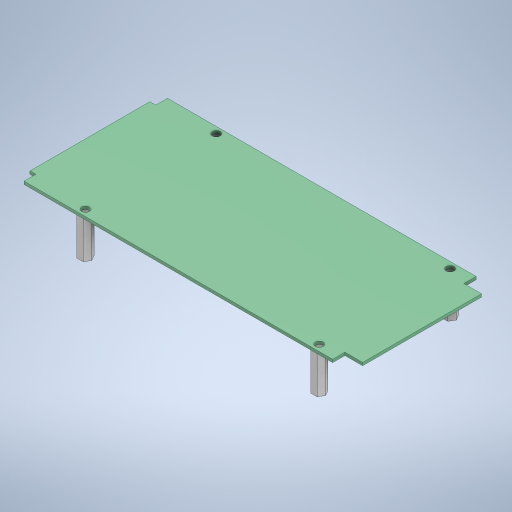
# Autodesk Inventor part: Tarjeta IC DC
Saved by Autodesk Inventor 2024.2 (Build 282272000, 272)
## iProperties
Created: 2024-08-27
Part Number: Tarjeta IC DC
Material: Phenolic Resin
Document SubType Name: Modeling
Designer: ja.restrepo1
Density: 1.38 g/cm^3
Appearance: Smooth - Dark Sea Green
Author: ja.restrepo1
Autodesk Inventor part; units mm, degrees
ref_plane "YZ Plane" through (0, 0, 0) normal (1, 0, 0) x (0, 1, 0)
ref_plane "XZ Plane" through (0, 0, 0) normal (0, 1, 0) x (-1, 0, 0)
ref_plane "XY Plane" through (0, 0, 0) normal (0, 0, 1) x (1, 0, 0)
sketch "Sketch1" plane through (0, 0, 0) normal (0, 1, 0) x (-1, 0, 0)
  line L0 (81.5, 36.5) -> (78.5, 36.5) construction
  line L1 (-78.5, 36.5) -> (-78.5, 30.25)
  line L2 (-78.5, -36.5) -> (78.5, -36.5)
  line L3 (81.5, -36.5) -> (81.5, -30.5) construction
  line L4 (-78.5, 30.25) -> (-87.5, 30.25)
  line L5 (-87.5, 30.25) -> (-87.5, -30.25)
  line L6 (-87.5, -30.25) -> (-78.5, -30.25)
  line L7 (-78.5, 30.25) -> (-78.5, -30.25) construction
  line L8 (-78.5, -30.25) -> (-78.5, -36.5)
  line L9 (81.5, 30.5) -> (78.5, 30.5)
  line L10 (78.5, 30.5) -> (78.5, 36.5)
  line L11 (78.5, 36.5) -> (-78.5, 36.5)
  line L12 (81.5, 30.5) -> (81.5, 36.5) construction
  line L13 (81.5, -30.5) -> (78.5, -30.5)
  line L14 (78.5, -30.5) -> (78.5, -36.5)
  line L15 (81.5, -30.5) -> (81.5, 30.5)
  line L16 (78.5, -36.5) -> (81.5, -36.5) construction
  circle A0 centre (-68.5, 33.25) radius 2
  circle A1 centre (-68.5, -33.25) radius 2
  circle A2 centre (50.5, -33.25) radius 2
  circle A3 centre (50.5, 33.25) radius 2
  line L17 (50.5, 33.25) -> (50.5, -33.25) construction
  line L18 (50.5, -33.25) -> (-68.5, -33.25) construction
  point P0 (0, 0)
  point P1 (-87.5, 0)
  point P2 (-78.5, 0)
  point P3 (81.5, 0)
  point P4 (0, -36.5)
  point P5 (50.5, 0)
  dimension "d3" = 9
  dimension "d4" = 60.5
  dimension "d6" = 3
  dimension "d7" = 6
  dimension "d8" = 160
  dimension "d12" = 3
  dimension "d13" = 6
  dimension "d14" = 61
  dimension "d15" = 4
  dimension "d16" = 66.5
  dimension "d17" = 119
  dimension "d18" = 19
  constraints: 38 end point, 13 parallel, 12 perpendicular, 6 horizontal alignment, 5 horizontal, 5 midpoint, 4 centre point, 3 equal radius, 3 vertical alignment, 1 point on line
  measures "d3" distance of L1.end L4.end
  measures "d4" distance of L4.end L5.end
  measures "d6" distance of L9.start L9.end
  measures "d7" distance of L9.end L0.end
  measures "d8" distance between parallel lines of L7 L3
  measures "d12" distance of L3.end L13.end
  measures "d13" distance of L13.end L2.end
  measures "d14" distance between parallel lines of L13 L9
  measures "d15" diameter of A0
  measures "d16" distance of L17.start L17.end
  measures "d17" distance of L17.end L18.end
  measures "d18" distance from line of L5 A0.centre
extrude "Tarjeta AD IC DC" add sketch "Sketch1" along normal mid plane 1.5
sketch "Sketch2" plane through (0, -0.75, 0) normal (0, 1, 0) x (1, 0, 0)
  circle A0 centre (-50.5, -33.25) radius 2 projected
  line L0 (-53.6754, -33.25) -> (-52.0877, -30.5)
  line L1 (-52.0877, -30.5) -> (-48.9123, -30.5)
  line L2 (-48.9123, -30.5) -> (-47.3246, -33.25)
  line L3 (-47.3246, -33.25) -> (-48.9123, -36)
  line L4 (-48.9123, -36) -> (-52.0877, -36)
  line L5 (-52.0877, -36) -> (-53.6754, -33.25)
  line L6 (-53.6754, 33.25) -> (-52.0877, 36)
  line L7 (-52.0877, 36) -> (-48.9123, 36)
  line L8 (-48.9123, 36) -> (-47.3246, 33.25)
  line L9 (-47.3246, 33.25) -> (-48.9123, 30.5)
  line L10 (-48.9123, 30.5) -> (-52.0877, 30.5)
  line L11 (-52.0877, 30.5) -> (-53.6754, 33.25)
  circle A1 centre (-50.5, 33.25) radius 2 projected
  line L12 (65.3246, -33.25) -> (66.9123, -30.5)
  line L13 (66.9123, -30.5) -> (70.0877, -30.5)
  line L14 (70.0877, -30.5) -> (71.6754, -33.25)
  line L15 (71.6754, -33.25) -> (70.0877, -36)
  line L16 (70.0877, -36) -> (66.9123, -36)
  line L17 (66.9123, -36) -> (65.3246, -33.25)
  line L18 (65.3246, 33.25) -> (66.9123, 36)
  line L19 (66.9123, 36) -> (70.0877, 36)
  line L20 (70.0877, 36) -> (71.6754, 33.25)
  line L21 (71.6754, 33.25) -> (70.0877, 30.5)
  line L22 (70.0877, 30.5) -> (66.9123, 30.5)
  line L23 (66.9123, 30.5) -> (65.3246, 33.25)
  circle A2 centre (68.5, 33.25) radius 2 projected
  circle A3 centre (68.5, -33.25) radius 2 projected
  point P0 (0, 0)
  dimension "d21" = 5.5
  dimension "d22" = 5.5
  dimension "d23" = 5.5
  dimension "d24" = 5.5
  constraints: 48 end point, 5 coincident, 4 horizontal, 2 vertical alignment, 52 other
  measures "d21" distance between parallel lines of L4 L1
  measures "d22" distance between parallel lines of L10 L7
  measures "d23" distance between parallel lines of L16 L13
  measures "d24" distance between parallel lines of L22 L19
extrude "Espaciador hexagonal" add sketch "Sketch2" against normal blind 19.5 separate body
body "Solid1"
